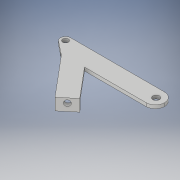
# Autodesk Inventor part: ventilador controladora_suportV
Saved by Autodesk Inventor 2019 (Build 230136000, 136)
## iProperties
Created: 2018-08-15
Part Number: ventilador controladora_suportV
Material: Genérico
Document SubType Name: Modeling
Designer: Albert Garangou Culebras
Density: 1 g/cm^3
Appearance: Valor por defecto
Author: Albert Garangou Culebras
Autodesk Inventor part; units mm, degrees
ref_plane "YZ Plane" through (0, 0, 0) normal (1, 0, 0) x (0, 1, 0)
ref_plane "XZ Plane" through (0, 0, 0) normal (0, 1, 0) x (-1, 0, 0)
ref_plane "XY Plane" through (0, 0, 0) normal (0, 0, 1) x (1, 0, 0)
sketch "Boceto1" plane through (0, 0, 0) normal (0, 1, 0) x (-1, 0, 0)
  line L0 (-2.031, 0) -> (-63, 0)
  line L1 (-65, -2) -> (-65, -8.0305)
  line L2 (-62.8998, -10.9676) -> (-2.0305, -10.9676)
  line L3 (0, -8.9987) -> (0, -2.031)
  line L4 (0, -8.9987) -> (0, -10.9676)
  line L5 (0, -10.9676) -> (-2.0305, -10.9676)
  line L6 (0, -2.031) -> (0, 0)
  line L7 (-65, -8.0305) -> (-65, -10.9676)
  line L8 (-65, -10.9676) -> (-62.8998, -10.9676)
  line L9 (-65, -2) -> (-65, 0)
  line L10 (-63, 0) -> (-65, 0)
  line L11 (0, 0) -> (-2.031, 0)
  dimension "d0" = 65
  constraints: 24 end point, 4 perpendicular, 4 point on line, 4 vertical, 3 horizontal
  measures "d0" distance of L6.end L9.end
extrude "Extrusión1" add sketch "Boceto1" along normal blind 3
sketch "Boceto2" plane through (0, 3, 0) normal (0, 1, 0) x (1, 0, 0)
  line L0 (0, 10.9676) -> (0, 0) projected
  circle A0 centre (5, 5.4838) radius 2
  line L1 (65, 0) -> (65, 10.9676) projected
  circle A1 centre (60, 5.4838) radius 2
  line L2 (65, 5.4838) -> (60, 5.4838)
  line L3 (0, 5.4838) -> (5, 5.4838)
  point P0 (0.1384, 8.9976)
  point P1 (0.0312, 2.0308)
  point P2 (65, 2)
  point P3 (65, 8.0305)
  dimension "d20" = 5
  dimension "d31" = 4
  dimension "d32" = 4
  constraints: 4 end point, 2 centre point, 2 horizontal, 1 coincident, 1 midpoint, 2 other
  measures "d20" distance of L2.start L2.end
  measures "d31" diameter of A0
  measures "d32" diameter of A1
extrude "Extrusión2" cut sketch "Boceto2" against normal blind 5
sketch "Boceto3" plane through (0, 3, 0) normal (0, 1, 0) x (1, 0, 0)
  circle A0 centre (5, 5.4838) radius 2 projected
  line L0 (5, 5.4838) -> (319.2562, 5.4838) construction
  line L1 (19.8683, -0.0721) -> (38.3706, -22.1223)
  line L2 (16.8683, -0.0721) -> (16.8078, 0)
  line L3 (11.4418, -7.1428) -> (5.4483, 0)
  line L4 (65, 0) -> (0, 0) projected
  line L5 (11.4418, -7.1428) -> (29.9441, -29.1929)
  line L6 (38.3706, -22.1223) -> (29.9441, -29.1929)
  line L7 (16.8078, 0) -> (19.8078, 0)
  line L8 (0, 0) -> (65, 0) projected
  dimension "d37" = 3
  constraints: 14 end point, 1 horizontal, 1 perpendicular, 1 point on line
  measures "d37" distance of L2.end L7.end
extrude "Extrusión3" add sketch "Boceto3" against normal blind 3
sketch "Boceto10" plane through (0, 3, 0) normal (0, 1, 0) x (1, 0, 0)
  line L0 (6.3645, 0) -> (-0.0991, 7.9201)
  line L1 (-0.0991, 7.9201) -> (0, 3)
  line L2 (2.4483, 0) -> (6.3645, 0)
  line L3 (65, 0) -> (0, 0) projected
  line L4 (2.4483, 0) -> (0, 0)
  line L5 (0, 0) -> (0, 3)
  constraints: 10 end point, 1 collinear, 1 perpendicular
extrude "Extrusión9" cut sketch "Boceto10" against normal blind 39
fillet "Empalme8" radius 5.48 2 edges at (65, 1.5, 0) (65, 1.5, -10.9676)
fillet "Empalme10" radius 3 2 edges at (0, 1.5, -7.7987) (0, 1.5, -10.9676)
sketch "Boceto11" plane through (0, 3, 0) normal (0, 1, 0) x (1, 0, 0)
  line L0 (0, 0) -> (0, 10.9676) projected
  line L1 (0, 3) -> (0, 0)
  line L2 (0, 0) -> (2.4483, 0)
  line L3 (2.4483, 0) -> (0, 3) projected
  line L4 (2.4483, 0) -> (0, 3)
  constraints: 6 end point, 2 collinear, 1 perpendicular
extrude "Extrusión10" cut sketch "Boceto11" against normal blind 57.75
sketch "Boceto13" plane through (0, 3, 0) normal (0, 1, 0) x (1, 0, 0)
  arc A0 (3.7344, 10.9676) -> (1.4102, 6.0708) centre (3.7344, 7.9676) ccw projected
  circle A1 centre (3.7344, 7.9676) radius 1.7
  point P0 (0, 0)
  dimension "d55" = 3.4
  constraints: 1 centre point, 1 coincident
  measures "d55" diameter of A1
extrude "Extrusión12" cut sketch "Boceto13" against normal blind 8
sketch "Boceto14" plane through (0, 3, 0) normal (0, 1, 0) x (1, 0, 0)
  line L0 (29.4887, -24.4468) -> (8.9754, 0)
  line L1 (59.52, 0) -> (6.3645, 0) projected
  line L2 (37.9152, -17.3762) -> (23.3349, 0)
  line L3 (37.9152, -17.3762) -> (29.4887, -24.4468)
  line L4 (23.3349, 0) -> (8.9754, 0)
  point P0 (0, 0)
  point P1 (37.6687, -20.1938)
  point P2 (10.2808, 0)
  constraints: 8 end point, 2 point on line, 1 collinear
extrude "Extrusión18" add sketch "Boceto14" against normal blind 2
sketch "Boceto19" plane through (0, 0, 0) normal (0, -1, 0) x (1, 0, 0)
  arc A0 (59.52, -10.9676) -> (65, -5.4876) centre (59.52, -5.4876) ccw projected
  arc A1 (1.4102, -6.0708) -> (3.7344, -10.9676) centre (3.7344, -7.9676) ccw projected
  line L0 (59.52, -10.9676) -> (3.7344, -10.9676)
  line L1 (6.3645, 0) -> (1.4102, -6.0708) projected
  line L2 (1.4102, -6.0708) -> (6.3645, 0)
  line L3 (6.3645, 0) -> (59.52, 0)
  arc A2 (59.52, -10.9676) -> (59.52, 0) centre (59.52, -5.4838) ccw
  line L4 (3.7344, -10.9676) -> (59.52, -10.9676) projected
  arc A3 (1.4102, -6.0708) -> (3.7344, -10.9676) centre (3.7344, -7.9676) ccw
  circle A4 centre (60, -5.4838) radius 2 projected
  circle A5 centre (60, -5.4838) radius 2
  circle A6 centre (3.7344, -7.9676) radius 1.7 projected
  circle A7 centre (3.7344, -7.9676) radius 1.6
  point P0 (0, 0)
  constraints: 6 end point, 5 tangent, 4 centre point, 4 point on circle, 2 coincident, 2 horizontal, 1 point on line
extrude "Extrusión19" cut sketch "Boceto19" against normal blind 1 contours L1 L3 A2 L0 A1
sketch "Boceto20" plane through (0, 1, 0) normal (0, -1, 0) x (1, 0, 0)
  line L0 (29.4887, 24.4468) -> (8.9754, 0) projected
  line L1 (1.4102, -6.0708) -> (6.3645, 0) projected
  line L2 (8.9754, 0) -> (1.4102, -6.0708)
  line L3 (6.3645, 0) -> (8.9754, 0) projected
  line L4 (8.9754, 0) -> (6, 0)
  line L5 (6, 0) -> (1.4102, -6.0708)
  point P0 (0, 0)
  constraints: 6 end point, 2 point on line, 1 collinear
extrude "Extrusión20" cut sketch "Boceto20" against normal blind 11.25 contours L1 L3 L2
sketch "Boceto21" plane through (0, 1, 0) normal (0, -1, 0) x (1, 0, 0)
  line L0 (29.4887, 24.4468) -> (8.9754, 0) projected
  line L1 (23.3349, 0) -> (8.9754, 0)
  line L2 (16.1551, 0) -> (22.9551, 0)
  line L3 (16.1551, 0) -> (9.3551, 0)
  line L4 (22.9551, 0) -> (37.6911, 17.5642)
  line L5 (37.9152, 17.3762) -> (29.4887, 24.4468) projected
  line L6 (37.6911, 17.5642) -> (37.9152, 17.3762)
  line L7 (23.3349, 0) -> (59.52, 0) projected
  line L8 (37.9152, 17.3762) -> (23.3349, 0)
  line L9 (23.3349, 0) -> (22.9551, 0)
  line L10 (9.3551, 0) -> (8.9754, 0)
  line L11 (9.3551, 0) -> (29.7116, 24.2599)
  line L12 (29.4887, 24.4468) -> (29.7116, 24.2599)
  point P0 (0, 0)
  dimension "d89" = 6.8
  dimension "d90" = 6.8
  constraints: 20 end point, 4 point on line, 3 collinear, 3 perpendicular, 1 horizontal, 1 midpoint
  measures "d89" distance of L2.start L2.end
  measures "d90" distance of L2.start L3.end
extrude "Extrusión21" cut sketch "Boceto21" against normal blind 11.25 contours L5 L11 L1 L0 | L5 L8 L1 L4
sketch "Boceto22" plane through (0, 1, 0) normal (0, -1, 0) x (1, 0, 0)
  line L0 (37.6911, 17.5642) -> (29.7116, 24.2599) projected
  line L1 (29.7116, 24.2599) -> (37.6911, 17.5642)
  line L2 (37.6911, 17.5642) -> (36.0843, 15.649)
  line L3 (22.9551, 0) -> (37.6911, 17.5642) projected
  line L4 (36.0843, 15.649) -> (28.1043, 22.3441)
  line L5 (28.1043, 22.3441) -> (29.7116, 24.2599)
  point P0 (0, 0)
  dimension "d94" = 2.5
  constraints: 8 end point, 2 perpendicular, 1 collinear, 1 point on line
  measures "d94" distance of L0.start L2.end
extrude "Extrusión22" add sketch "Boceto22" along normal blind 5
sketch "Boceto23" plane through (37.6911, -4, 17.5642) normal (0.6427876, 0, 0.7660444) x (0.7660444, 0, -0.6427876)
  line L0 (-10.4166, 7) -> (0, 7) projected
  line L1 (-5.2083, 7) -> (-5.2081, 0)
  line L2 (-10.4164, 0) -> (0.0002, 0) projected
  line L3 (0.0002, 5) -> (-10.4164, 5) projected
  line L4 (-5.2081, 5) -> (-5.2083, 6)
  line L5 (-5.2083, 6) -> (-5.2082, 2.6)
  circle A0 centre (-5.2082, 4.3) radius 1.7
  point P0 (-17.583, 4)
  dimension "d97" = 3.4
  constraints: 6 end point, 4 midpoint, 2 point on line, 3 other
  measures "d97" distance of L4.end L5.end
extrude "Extrusión23" cut sketch "Boceto23" against normal blind 10
sketch "Boceto26" plane through (0, 1, 0) normal (0, -1, 0) x (1, 0, 0)
  line L0 (33.3965, 17.904) -> (30.7918, 20.0892) projected
  line L1 (32.0942, 18.9966) -> (29.7959, 20.9248)
  line L2 (29.7959, 20.9248) -> (34.3925, 17.0684)
  line L3 (36.0843, 15.649) -> (33.281, 18.0009) projected
  line L4 (34.3925, 17.0684) -> (31.1788, 13.2379)
  line L5 (31.1788, 13.2379) -> (26.5822, 17.0943)
  line L6 (26.5822, 17.0943) -> (29.7959, 20.9248)
  point P0 (0, 0)
  point P1 (30.9074, 19.9923)
  dimension "d103" = 3
  dimension "d104" = 6
  dimension "d106" = 5
  constraints: 10 end point, 3 perpendicular, 1 collinear, 1 midpoint, 1 point on line
  measures "d103" distance of L1.start L1.end
  measures "d104" distance of L1.end L2.end
  measures "d106" distance of L2.end L4.end
extrude "Extrusión25" cut sketch "Boceto26" against normal blind 0.9
